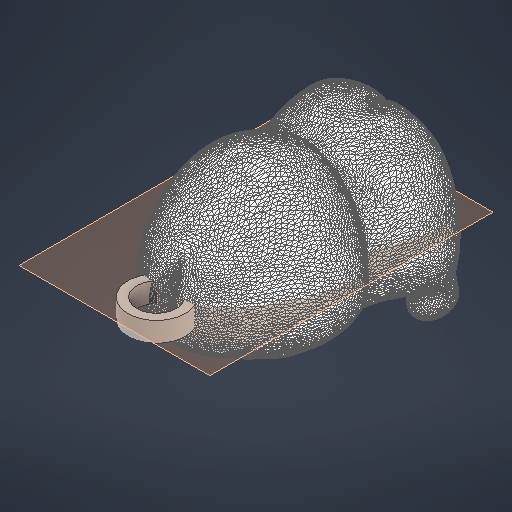
# Autodesk Inventor part: TK_Ding_Ding
Saved by Autodesk Inventor 2025.3 (Build 293356030, 356C)
## iProperties
Created: 2025-10-03
Part Number: TK_Ding_Ding
Material: Generic
Document SubType Name: Modeling
Designer: yo
Density: 1 g/cm^3
Appearance: Default
Author: yo
Autodesk Inventor part; units mm, degrees
ref_plane "YZ Plane" through (0, 0, 0) normal (1, 0, 0) x (0, 1, 0)
ref_plane "XY Plane" through (0, 0, 0) normal (0, 0, 1) x (1, 0, 0)
sketch "Sketch1" plane through (0, 0, 0) normal (0, 1, 0) x (-1, 0, 0)
  line L0 (4.8437, 49.0141) -> (2.3437, 49.0141)
  line L1 (-6.4563, 49.0141) -> (-3.9563, 49.0141)
  arc A0 (2.3437, 49.0141) -> (-3.9563, 49.0141) centre (-0.8063, 52.2277) ccw
  arc A1 (4.8437, 49.0141) -> (-6.4563, 49.0141) centre (-0.8063, 52.2277) ccw
  point P0 (0, 0)
  dimension "d0" = 2.5
  dimension "d2" = 4.5
  dimension "d3" = 6.5
  constraints: 4 end point, 4 point on circle, 2 centre point, 2 collinear, 1 coincident, 1 horizontal
  measures "d0" distance of L0.start L0.end
  measures "d2" radius of A0
  measures "d3" radius of A1
extrude "Extrusion1" add sketch "Sketch1" against normal blind 4.5
body "Solid1"
